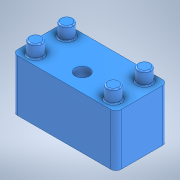
# Autodesk Inventor part: Foot_Spacer
Saved by Autodesk Inventor 2021 (Build 250183000, 183)
## iProperties
Created: 2021-05-18
Part Number: Foot_Spacer
Material: Generic
Document SubType Name: Modeling
Designer: Jorian Brusind
Density: 1 g/cm^3
Appearance: Cyan
Author: Jorian Brusind
Autodesk Inventor part; units mm, degrees
ref_plane "YZ Plane" through (0, 0, 0) normal (1, 0, 0) x (0, 1, 0)
ref_plane "XZ Plane" through (0, 0, 0) normal (0, 1, 0) x (-1, 0, 0)
ref_plane "XY Plane" through (0, 0, 0) normal (0, 0, 1) x (1, 0, 0)
sketch "Sketch1" plane through (0, 0, 0) normal (0, 1, 0) x (-1, 0, 0)
  line L0 (0, 0) -> (40, 0)
  line L1 (40, 0) -> (40, -20)
  line L2 (40, -20) -> (0, -20)
  line L3 (0, -20) -> (0, 0)
  dimension "d0" = 40
  dimension "d1" = 20
  constraints: 8 end point, 2 parallel, 1 horizontal, 1 perpendicular
  measures "d0" distance of L1.end L2.end
  measures "d1" distance of L0.end L1.end
extrude "Extrusion1" add sketch "Sketch1" along normal blind 20
sketch "Sketch2" plane through (0, 20, 0) normal (0, 1, 0) x (1, 0, 0)
  circle A0 centre (-35, 4) radius 2.5
  line L0 (-40, 20) -> (-40, 0) projected
  line L1 (-40, 0) -> (0, 0) projected
  circle A1 centre (-35, 16) radius 2.5
  circle A2 centre (-5, 4) radius 2.5
  circle A3 centre (-5, 16) radius 2.5
  dimension "d4" = 5
  dimension "d5" = 5
  dimension "d6" = 4
  dimension "d9" = 12
  dimension "d12" = 30
  constraints: 4 centre point, 1 horizontal, 1 vertical, 6 other
  measures "d4" diameter of A0
  measures "d5" distance from line of L0 A0.centre
  measures "d6" distance from line of L1 A0.centre
  measures "d9" distance of A0.centre A1.centre
  measures "d12" distance of A0.centre A2.centre
extrude "Extrusion2" add sketch "Sketch2" along normal blind 5
fillet "Fillet1" radius 0.5 8 edges at (-37.5, 20, -4) (-7.5, 20, -4) (-7.5, 20, -16) (-37.5, 20, -16) (-37.5, 25, -16) (-7.5, 25, -16) (-7.5, 25, -4) (-37.5, 25, -4) curvature continuous yes
sketch "Sketch3" plane through (0, 0, 0) normal (0, -1, 0) x (1, 0, 0)
  circle A0 centre (-20, -7) radius 2.75
  line L0 (0, 0) -> (0, -20) projected
  line L1 (-40, 0) -> (0, 0) projected
  dimension "d18" = 5.5
  dimension "d19" = 20
  dimension "d20" = 7
  constraints: 1 centre point
  measures "d18" diameter of A0
  measures "d19" distance from line of L0 A0.centre
  measures "d20" distance from line of L1 A0.centre
extrude "Extrusion3" cut sketch "Sketch3" against normal through all
sketch "Sketch4" plane through (0, 0, 0) normal (0, -1, 0) x (1, 0, 0)
  circle A0 centre (-20, -7) radius 2.75 projected
  line L0 (-15.3812, -7) -> (-17.6906, -11)
  line L1 (-17.6906, -11) -> (-22.3094, -11)
  line L2 (-22.3094, -11) -> (-24.6188, -7)
  line L3 (-24.6188, -7) -> (-22.3094, -3)
  line L4 (-22.3094, -3) -> (-17.6906, -3)
  line L5 (-17.6906, -3) -> (-15.3812, -7)
  line L6 (0, 0) -> (0, -20) projected
  dimension "d23" = 8
  dimension "d24" = 90
  constraints: 12 end point, 1 coincident, 13 other
  measures "d23" distance between parallel lines of L1 L4
  measures "d24" angle of L6 L1
extrude "Extrusion4" cut sketch "Sketch4" against normal blind 4
sketch "Sketch5" plane through (0, 0, 0) normal (0, -1, 0) x (1, 0, 0)
  circle A0 centre (-5, -4) radius 2 projected
  circle A1 centre (-5, -4) radius 2.75
  line L0 (0, 0) -> (0, -20) projected
  line L1 (0, 0) -> (0, -20)
  line L2 (-40, 0) -> (0, 0) projected
  line L3 (0, 0) -> (-40, 0)
  circle A2 centre (-5, -16) radius 2.75
  circle A3 centre (-35, -4) radius 2.75
  circle A4 centre (-35, -16) radius 2.75
  point P0 (-3, -4)
  dimension "d27" = 5.5
  dimension "d30" = 12
  dimension "d33" = 30
  constraints: 4 centre point, 4 end point, 2 vertical, 1 coincident, 1 collinear, 1 horizontal, 1 horizontal alignment, 6 other
  measures "d27" diameter of A1
  measures "d30" distance of A1.centre A2.centre
  measures "d33" distance of A1.centre A3.centre
extrude "Extrusion5" cut sketch "Sketch5" against normal blind 5.5 contours A0 | A1 | A2 | A3 | A4
fillet "Fillet2" radius 2 4 edges at (-40, 10, 0) (0, 10, 0) (-40, 10, -20) (0, 10, -20)
body "Solid1"
